Autodesk Fusion 360 part; units mm, degrees
(part 2 of 6)
  spline S13 degree 5 poles (-24.4636, 3.0462) (-24.4632, 3.0438) (-24.4623, 3.0389) (-24.4609, 3.0317) (-24.4591, 3.022) (-24.4568, 3.0099) (-24.4544, 2.9979) (-24.4519, 2.9859) (-24.4494, 2.9739) (-24.4468, 2.962) (-24.4442, 2.9501) (-24.4415, 2.9383) (-24.4387, 2.9265) (-24.4359, 2.9147) (-24.4331, 2.903) (-24.4301, 2.8914) (-24.4271, 2.8797) (-24.4241, 2.8681) (-24.421, 2.8566) (-24.4178, 2.8451) (-24.4146, 2.8336) (-24.4113, 2.8222) (-24.4079, 2.8108) (-24.4045, 2.7995) (-24.4011, 2.7882) (-24.3975, 2.777) (-24.3939, 2.7658) (-24.3903, 2.7547) (-24.3866, 2.7436) (-24.3828, 2.7325) (-24.379, 2.7215) (-24.3751, 2.7106) (-24.3711, 2.6997) (-24.3671, 2.6888) (-24.363, 2.678) (-24.3588, 2.6673) (-24.3546, 2.6566) (-24.3504, 2.646) (-24.346, 2.6354) (-24.3416, 2.6249) (-24.3372, 2.6144) (-24.3326, 2.604) (-24.328, 2.5936) (-24.3234, 2.5834) (-24.3186, 2.5731) (-24.3138, 2.5629) (-24.309, 2.5528) (-24.304, 2.5428) (-24.299, 2.5328) (-24.294, 2.5229) (-24.2888, 2.513) (-24.2836, 2.5032) (-24.2783, 2.4935) (-24.2729, 2.4839) (-24.2675, 2.4743) (-24.262, 2.4648) (-24.2564, 2.4554) (-24.2507, 2.446) (-24.245, 2.4368) (-24.2392, 2.4276) (-24.2333, 2.4185) (-24.2273, 2.4095) (-24.2211, 2.4006) (-24.2149, 2.3919) (-24.2085, 2.3832) (-24.2021, 2.3747) (-24.1956, 2.3662) (-24.1891, 2.3577) (-24.1825, 2.3494) (-24.1757, 2.3412) (-24.1687, 2.3333) (-24.1629, 2.3272) (-24.1583, 2.3228) (-24.1552, 2.32) (-24.1536, 2.3186) knots -1 -1 -1 -1 -1 -1 -0.98571429 -0.97142857 -0.95714286 -0.94285714 -0.92857143 -0.91428571 -0.9 -0.88571429 -0.87142857 -0.85714286 -0.84285714 -0.82857143 -0.81428571 -0.8 -0.78571429 -0.77142857 -0.75714286 -0.74285714 -0.72857143 -0.71428571 -0.7 -0.68571429 -0.67142857 -0.65714286 -0.64285714 -0.62857143 -0.61428571 -0.6 -0.58571429 -0.57142857 -0.55714286 -0.54285714 -0.52857143 -0.51428571 -0.5 -0.48571429 -0.47142857 -0.45714286 -0.44285714 -0.42857143 -0.41428571 -0.4 -0.38571429 -0.37142857 -0.35714286 -0.34285714 -0.32857143 -0.31428571 -0.3 -0.28571429 -0.27142857 -0.25714286 -0.24285714 -0.22857143 -0.21428571 -0.2 -0.18571429 -0.17142857 -0.15714286 -0.14285714 -0.12857143 -0.11428571 -0.1 -0.08571429 -0.07142857 -0.05714286 -0.04285714 -0.02857143 -0.01428571 0 0 0 0 0 0
  line L13 (-24.1536, 2.3186) -> (-24.0344, 2.2145)
  arc A27 (-24.0078, 1.9414) -> (-24.0344, 2.2145) centre (-24.166, 2.0639) ccw
  arc A28 (-24.0078, 1.9414) -> (-24.1214, 1.7852) centre (-21.5, 0) ccw
  arc A29 (-24.3893, 1.726) -> (-24.1214, 1.7852) centre (-24.2867, 1.8977) ccw
  line L14 (-24.3893, 1.726) -> (-24.5251, 1.8072)
  spline S14 degree 5 poles (-24.5251, 1.8072) (-24.527, 1.8083) (-24.5306, 1.8104) (-24.5362, 1.8134) (-24.5438, 1.8171) (-24.5535, 1.8213) (-24.5633, 1.8252) (-24.5733, 1.8289) (-24.5833, 1.8325) (-24.5934, 1.8361) (-24.6036, 1.8395) (-24.6137, 1.8429) (-24.624, 1.8461) (-24.6343, 1.8492) (-24.6447, 1.8522) (-24.6552, 1.855) (-24.6658, 1.8577) (-24.6764, 1.8602) (-24.687, 1.8627) (-24.6977, 1.8651) (-24.7084, 1.8674) (-24.7192, 1.8697) (-24.73, 1.8718) (-24.7409, 1.8738) (-24.7518, 1.8758) (-24.7628, 1.8776) (-24.7738, 1.8794) (-24.7848, 1.881) (-24.7959, 1.8826) (-24.807, 1.8841) (-24.8182, 1.8855) (-24.8294, 1.8869) (-24.8406, 1.8881) (-24.8519, 1.8893) (-24.8632, 1.8904) (-24.8745, 1.8914) (-24.8859, 1.8923) (-24.8973, 1.8932) (-24.9087, 1.894) (-24.9202, 1.8947) (-24.9317, 1.8953) (-24.9432, 1.8959) (-24.9548, 1.8963) (-24.9664, 1.8967) (-24.978, 1.8971) (-24.9896, 1.8973) (-25.0013, 1.8975) (-25.013, 1.8976) (-25.0247, 1.8976) (-25.0365, 1.8976) (-25.0482, 1.8975) (-25.06, 1.8973) (-25.0719, 1.897) (-25.0837, 1.8967) (-25.0956, 1.8963) (-25.1075, 1.8958) (-25.1194, 1.8953) (-25.1313, 1.8947) (-25.1433, 1.894) (-25.1553, 1.8932) (-25.1673, 1.8924) (-25.1793, 1.8915) (-25.1914, 1.8906) (-25.2035, 1.8895) (-25.2156, 1.8884) (-25.2277, 1.8873) (-25.2398, 1.8861) (-25.2519, 1.8848) (-25.2641, 1.8834) (-25.2763, 1.8819) (-25.2885, 1.8804) (-25.2983, 1.8792) (-25.3056, 1.8782) (-25.3105, 1.8776) (-25.3129, 1.8772) knots 0 0 0 0 0 0 0.01428571 0.02857143 0.04285714 0.05714286 0.07142857 0.08571429 0.1 0.11428571 0.12857143 0.14285714 0.15714286 0.17142857 0.18571429 0.2 0.21428571 0.22857143 0.24285714 0.25714286 0.27142857 0.28571429 0.3 0.31428571 0.32857143 0.34285714 0.35714286 0.37142857 0.38571429 0.4 0.41428571 0.42857143 0.44285714 0.45714286 0.47142857 0.48571429 0.5 0.51428571 0.52857143 0.54285714 0.55714286 0.57142857 0.58571429 0.6 0.61428571 0.62857143 0.64285714 0.65714286 0.67142857 0.68571429 0.7 0.71428571 0.72857143 0.74285714 0.75714286 0.77142857 0.78571429 0.8 0.81428571 0.82857143 0.84285714 0.85714286 0.87142857 0.88571429 0.9 0.91428571 0.92857143 0.94285714 0.95714286 0.97142857 0.98571429 1 1 1 1 1 1
  arc A30 (-25.3129, 1.8772) -> (-25.4464, 1.5775) centre (-21.5, 0) ccw
  spline S15 degree 5 poles (-25.4464, 1.5775) (-25.445, 1.5754) (-25.4422, 1.5713) (-25.438, 1.5652) (-25.4324, 1.5571) (-25.4254, 1.5471) (-25.4183, 1.537) (-25.4112, 1.5271) (-25.404, 1.5172) (-25.3968, 1.5074) (-25.3896, 1.4976) (-25.3823, 1.4879) (-25.375, 1.4782) (-25.3676, 1.4686) (-25.3603, 1.4591) (-25.3528, 1.4496) (-25.3454, 1.4402) (-25.3379, 1.4308) (-25.3303, 1.4216) (-25.3228, 1.4123) (-25.3151, 1.4032) (-25.3075, 1.3941) (-25.2998, 1.3851) (-25.2921, 1.3761) (-25.2843, 1.3672) (-25.2765, 1.3584) (-25.2687, 1.3496) (-25.2608, 1.3409) (-25.2529, 1.3323) (-25.245, 1.3237) (-25.237, 1.3153) (-25.229, 1.3068) (-25.2209, 1.2985) (-25.2129, 1.2902) (-25.2047, 1.282) (-25.1966, 1.2739) (-25.1884, 1.2659) (-25.1802, 1.2579) (-25.1719, 1.25) (-25.1636, 1.2422) (-25.1553, 1.2344) (-25.1469, 1.2267) (-25.1385, 1.2192) (-25.13, 1.2116) (-25.1215, 1.2042) (-25.113, 1.1969) (-25.1045, 1.1896) (-25.0959, 1.1824) (-25.0872, 1.1753) (-25.0786, 1.1683) (-25.0699, 1.1614) (-25.0611, 1.1546) (-25.0523, 1.1479) (-25.0435, 1.1413) (-25.0346, 1.1348) (-25.0257, 1.1283) (-25.0168, 1.122) (-25.0078, 1.1157) (-24.9988, 1.1096) (-24.9898, 1.1036) (-24.9807, 1.0976) (-24.9715, 1.0919) (-24.9623, 1.0863) (-24.953, 1.0808) (-24.9437, 1.0755) (-24.9344, 1.0703) (-24.925, 1.0652) (-24.9156, 1.0601) (-24.9062, 1.0552) (-24.8967, 1.0505) (-24.887, 1.0461) (-24.8792, 1.0429) (-24.8733, 1.0408) (-24.8693, 1.0395) (-24.8672, 1.0389) knots -1 -1 -1 -1 -1 -1 -0.98571429 -0.97142857 -0.95714286 -0.94285714 -0.92857143 -0.91428571 -0.9 -0.88571429 -0.87142857 -0.85714286 -0.84285714 -0.82857143 -0.81428571 -0.8 -0.78571429 -0.77142857 -0.75714286 -0.74285714 -0.72857143 -0.71428571 -0.7 -0.68571429 -0.67142857 -0.65714286 -0.64285714 -0.62857143 -0.61428571 -0.6 -0.58571429 -0.57142857 -0.55714286 -0.54285714 -0.52857143 -0.51428571 -0.5 -0.48571429 -0.47142857 -0.45714286 -0.44285714 -0.42857143 -0.41428571 -0.4 -0.38571429 -0.37142857 -0.35714286 -0.34285714 -0.32857143 -0.31428571 -0.3 -0.28571429 -0.27142857 -0.25714286 -0.24285714 -0.22857143 -0.21428571 -0.2 -0.18571429 -0.17142857 -0.15714286 -0.14285714 -0.12857143 -0.11428571 -0.1 -0.08571429 -0.07142857 -0.05714286 -0.04285714 -0.02857143 -0.01428571 0 0 0 0 0 0
  line L15 (-24.8672, 1.0389) -> (-24.716, 0.9922)
  arc A31 (-24.5807, 0.7536) -> (-24.716, 0.9922) centre (-24.7749, 0.8011) ccw
  arc A32 (-24.5807, 0.7536) -> (-24.6208, 0.5646) centre (-21.5, 0) ccw
  arc A33 (-24.8415, 0.4016) -> (-24.6208, 0.5646) centre (-24.8176, 0.6002) ccw
  line L16 (-24.8415, 0.4016) -> (-24.9987, 0.4205)
  spline S16 degree 5 poles (-24.9987, 0.4205) (-25.0008, 0.4208) (-25.005, 0.4212) (-25.0113, 0.4217) (-25.0197, 0.422) (-25.0303, 0.4219) (-25.0409, 0.4214) (-25.0515, 0.4208) (-25.0621, 0.42) (-25.0728, 0.4191) (-25.0834, 0.4181) (-25.0941, 0.4171) (-25.1048, 0.4159) (-25.1155, 0.4145) (-25.1262, 0.413) (-25.1369, 0.4113) (-25.1476, 0.4094) (-25.1584, 0.4075) (-25.1691, 0.4054) (-25.1799, 0.4033) (-25.1906, 0.401) (-25.2013, 0.3987) (-25.2121, 0.3962) (-25.2229, 0.3936) (-25.2336, 0.391) (-25.2444, 0.3882) (-25.2552, 0.3853) (-25.2659, 0.3824) (-25.2767, 0.3793) (-25.2875, 0.3761) (-25.2982, 0.3729) (-25.309, 0.3696) (-25.3198, 0.3661) (-25.3305, 0.3626) (-25.3413, 0.359) (-25.3521, 0.3554) (-25.3629, 0.3516) (-25.3736, 0.3477) (-25.3844, 0.3438) (-25.3951, 0.3398) (-25.4059, 0.3357) (-25.4167, 0.3315) (-25.4274, 0.3272) (-25.4381, 0.3229) (-25.4489, 0.3184) (-25.4596, 0.3139) (-25.4704, 0.3093) (-25.4811, 0.3047) (-25.4918, 0.2999) (-25.5025, 0.2951) (-25.5132, 0.2902) (-25.5239, 0.2853) (-25.5346, 0.2802) (-25.5453, 0.2751) (-25.556, 0.2699) (-25.5667, 0.2646) (-25.5774, 0.2593) (-25.588, 0.2539) (-25.5987, 0.2484) (-25.6093, 0.2428) (-25.62, 0.2372) (-25.6306, 0.2315) (-25.6412, 0.2257) (-25.6518, 0.2199) (-25.6624, 0.2139) (-25.673, 0.2079) (-25.6836, 0.2019) (-25.6942, 0.1958) (-25.7047, 0.1896) (-25.7153, 0.1833) (-25.7258, 0.177) (-25.7342, 0.1718) (-25.7405, 0.168) (-25.7447, 0.1654) (-25.7468, 0.1641) knots 0 0 0 0 0 0 0.01428571 0.02857143 0.04285714 0.05714286 0.07142857 0.08571429 0.1 0.11428571 0.12857143 0.14285714 0.15714286 0.17142857 0.18571429 0.2 0.21428571 0.22857143 0.24285714 0.25714286 0.27142857 0.28571429 0.3 0.31428571 0.32857143 0.34285714 0.35714286 0.37142857 0.38571429 0.4 0.41428571 0.42857143 0.44285714 0.45714286 0.47142857 0.48571429 0.5 0.51428571 0.52857143 0.54285714 0.55714286 0.57142857 0.58571429 0.6 0.61428571 0.62857143 0.64285714 0.65714286 0.67142857 0.68571429 0.7 0.71428571 0.72857143 0.74285714 0.75714286 0.77142857 0.78571429 0.8 0.81428571 0.82857143 0.84285714 0.85714286 0.87142857 0.88571429 0.9 0.91428571 0.92857143 0.94285714 0.95714286 0.97142857 0.98571429 1 1 1 1 1 1
  arc A34 (-25.7468, 0.1641) -> (-25.7468, -0.1641) centre (-21.5, 0) ccw
  spline S17 degree 5 poles (-25.7468, -0.1641) (-25.7447, -0.1654) (-25.7405, -0.168) (-25.7342, -0.1718) (-25.7258, -0.177) (-25.7153, -0.1833) (-25.7047, -0.1896) (-25.6942, -0.1958) (-25.6836, -0.2019) (-25.673, -0.2079) (-25.6624, -0.2139) (-25.6518, -0.2199) (-25.6412, -0.2257) (-25.6306, -0.2315) (-25.62, -0.2372) (-25.6093, -0.2428) (-25.5987, -0.2484) (-25.588, -0.2539) (-25.5774, -0.2593) (-25.5667, -0.2646) (-25.556, -0.2699) (-25.5453, -0.2751) (-25.5346, -0.2802) (-25.5239, -0.2853) (-25.5132, -0.2902) (-25.5025, -0.2951) (-25.4918, -0.2999) (-25.4811, -0.3047) (-25.4704, -0.3093) (-25.4596, -0.3139) (-25.4489, -0.3184) (-25.4381, -0.3229) (-25.4274, -0.3272) (-25.4167, -0.3315) (-25.4059, -0.3357) (-25.3951, -0.3398) (-25.3844, -0.3438) (-25.3736, -0.3477) (-25.3629, -0.3516) (-25.3521, -0.3554) (-25.3413, -0.359) (-25.3305, -0.3626) (-25.3198, -0.3661) (-25.309, -0.3696) (-25.2982, -0.3729) (-25.2875, -0.3761) (-25.2767, -0.3793) (-25.2659, -0.3824) (-25.2552, -0.3853) (-25.2444, -0.3882) (-25.2336, -0.391) (-25.2229, -0.3936) (-25.2121, -0.3962) (-25.2013, -0.3987) (-25.1906, -0.401) (-25.1799, -0.4033) (-25.1691, -0.4054) (-25.1584, -0.4075) (-25.1476, -0.4094) (-25.1369, -0.4113) (-25.1262, -0.413) (-25.1155, -0.4145) (-25.1048, -0.4159) (-25.0941, -0.4171) (-25.0834, -0.4181) (-25.0728, -0.4191) (-25.0621, -0.42) (-25.0515, -0.4208) (-25.0409, -0.4214) (-25.0303, -0.4219) (-25.0197, -0.422) (-25.0113, -0.4217) (-25.005, -0.4212) (-25.0008, -0.4208) (-24.9987, -0.4205) knots -1 -1 -1 -1 -1 -1 -0.98571429 -0.97142857 -0.95714286 -0.94285714 -0.92857143 -0.91428571 -0.9 -0.88571429 -0.87142857 -0.85714286 -0.84285714 -0.82857143 -0.81428571 -0.8 -0.78571429 -0.77142857 -0.75714286 -0.74285714 -0.72857143 -0.71428571 -0.7 -0.68571429 -0.67142857 -0.65714286 -0.64285714 -0.62857143 -0.61428571 -0.6 -0.58571429 -0.57142857 -0.55714286 -0.54285714 -0.52857143 -0.51428571 -0.5 -0.48571429 -0.47142857 -0.45714286 -0.44285714 -0.42857143 -0.41428571 -0.4 -0.38571429 -0.37142857 -0.35714286 -0.34285714 -0.32857143 -0.31428571 -0.3 -0.28571429 -0.27142857 -0.25714286 -0.24285714 -0.22857143 -0.21428571 -0.2 -0.18571429 -0.17142857 -0.15714286 -0.14285714 -0.12857143 -0.11428571 -0.1 -0.08571429 -0.07142857 -0.05714286 -0.04285714 -0.02857143 -0.01428571 0 0 0 0 0 0
  line L17 (-24.9987, -0.4205) -> (-24.8415, -0.4016)
  arc A35 (-24.6208, -0.5646) -> (-24.8415, -0.4016) centre (-24.8176, -0.6002) ccw
  arc A36 (-24.6208, -0.5646) -> (-24.5807, -0.7536) centre (-21.5, 0) ccw
  arc A37 (-24.716, -0.9922) -> (-24.5807, -0.7536) centre (-24.7749, -0.8011) ccw
  line L18 (-24.716, -0.9922) -> (-24.8672, -1.0389)
  spline S18 degree 5 poles (-24.8672, -1.0389) (-24.8693, -1.0395) (-24.8733, -1.0408) (-24.8792, -1.0429) (-24.887, -1.0461) (-24.8967, -1.0505) (-24.9062, -1.0552) (-24.9156, -1.0601) (-24.925, -1.0652) (-24.9344, -1.0703) (-24.9437, -1.0755) (-24.953, -1.0808) (-24.9623, -1.0863) (-24.9715, -1.0919) (-24.9807, -1.0976) (-24.9898, -1.1036) (-24.9988, -1.1096) (-25.0078, -1.1157) (-25.0168, -1.122) (-25.0257, -1.1283) (-25.0346, -1.1348) (-25.0435, -1.1413) (-25.0523, -1.1479) (-25.0611, -1.1546) (-25.0699, -1.1614) (-25.0786, -1.1683) (-25.0872, -1.1753) (-25.0959, -1.1824) (-25.1045, -1.1896) (-25.113, -1.1969) (-25.1215, -1.2042) (-25.13, -1.2116) (-25.1385, -1.2192) (-25.1469, -1.2267) (-25.1553, -1.2344) (-25.1636, -1.2422) (-25.1719, -1.25) (-25.1802, -1.2579) (-25.1884, -1.2659) (-25.1966, -1.2739) (-25.2047, -1.282) (-25.2129, -1.2902) (-25.2209, -1.2985) (-25.229, -1.3068) (-25.237, -1.3153) (-25.245, -1.3237) (-25.2529, -1.3323) (-25.2608, -1.3409) (-25.2687, -1.3496) (-25.2765, -1.3584) (-25.2843, -1.3672) (-25.2921, -1.3761) (-25.2998, -1.3851) (-25.3075, -1.3941) (-25.3151, -1.4032) (-25.3228, -1.4123) (-25.3303, -1.4216) (-25.3379, -1.4308) (-25.3454, -1.4402) (-25.3528, -1.4496) (-25.3603, -1.4591) (-25.3676, -1.4686) (-25.375, -1.4782) (-25.3823, -1.4879) (-25.3896, -1.4976) (-25.3968, -1.5074) (-25.404, -1.5172) (-25.4112, -1.5271) (-25.4183, -1.537) (-25.4254, -1.5471) (-25.4324, -1.5571) (-25.438, -1.5652) (-25.4422, -1.5713) (-25.445, -1.5754) (-25.4464, -1.5775) knots 0 0 0 0 0 0 0.01428571 0.02857143 0.04285714 0.05714286 0.07142857 0.08571429 0.1 0.11428571 0.12857143 0.14285714 0.15714286 0.17142857 0.18571429 0.2 0.21428571 0.22857143 0.24285714 0.25714286 0.27142857 0.28571429 0.3 0.31428571 0.32857143 0.34285714 0.35714286 0.37142857 0.38571429 0.4 0.41428571 0.42857143 0.44285714 0.45714286 0.47142857 0.48571429 0.5 0.51428571 0.52857143 0.54285714 0.55714286 0.57142857 0.58571429 0.6 0.61428571 0.62857143 0.64285714 0.65714286 0.67142857 0.68571429 0.7 0.71428571 0.72857143 0.74285714 0.75714286 0.77142857 0.78571429 0.8 0.81428571 0.82857143 0.84285714 0.85714286 0.87142857 0.88571429 0.9 0.91428571 0.92857143 0.94285714 0.95714286 0.97142857 0.98571429 1 1 1 1 1 1
  arc A38 (-25.4464, -1.5775) -> (-25.3129, -1.8772) centre (-21.5, 0) ccw
  spline S19 degree 5 poles (-25.3129, -1.8772) (-25.3105, -1.8776) (-25.3056, -1.8782) (-25.2983, -1.8792) (-25.2885, -1.8804) (-25.2763, -1.8819) (-25.2641, -1.8834) (-25.2519, -1.8848) (-25.2398, -1.8861) (-25.2277, -1.8873) (-25.2156, -1.8884) (-25.2035, -1.8895) (-25.1914, -1.8906) (-25.1793, -1.8915) (-25.1673, -1.8924) (-25.1553, -1.8932) (-25.1433, -1.894) (-25.1313, -1.8947) (-25.1194, -1.8953) (-25.1075, -1.8958) (-25.0956, -1.8963) (-25.0837, -1.8967) (-25.0719, -1.897) (-25.06, -1.8973) (-25.0482, -1.8975) (-25.0365, -1.8976) (-25.0247, -1.8976) (-25.013, -1.8976) (-25.0013, -1.8975) (-24.9896, -1.8973) (-24.978, -1.8971) (-24.9664, -1.8967) (-24.9548, -1.8963) (-24.9432, -1.8959) (-24.9317, -1.8953) (-24.9202, -1.8947) (-24.9087, -1.894) (-24.8973, -1.8932) (-24.8859, -1.8923) (-24.8745, -1.8914) (-24.8632, -1.8904) (-24.8519, -1.8893) (-24.8406, -1.8881) (-24.8294, -1.8869) (-24.8182, -1.8855) (-24.807, -1.8841) (-24.7959, -1.8826) (-24.7848, -1.881) (-24.7738, -1.8794) (-24.7628, -1.8776) (-24.7518, -1.8758) (-24.7409, -1.8738) (-24.73, -1.8718) (-24.7192, -1.8697) (-24.7084, -1.8674) (-24.6977, -1.8651) (-24.687, -1.8627) (-24.6764, -1.8602) (-24.6658, -1.8577) (-24.6552, -1.855) (-24.6447, -1.8522) (-24.6343, -1.8492) (-24.624, -1.8461) (-24.6137, -1.8429) (-24.6036, -1.8395) (-24.5934, -1.8361) (-24.5833, -1.8325) (-24.5733, -1.8289) (-24.5633, -1.8252) (-24.5535, -1.8213) (-24.5438, -1.8171) (-24.5362, -1.8134) (-24.5306, -1.8104) (-24.527, -1.8083) (-24.5251, -1.8072) knots -1 -1 -1 -1 -1 -1 -0.98571429 -0.97142857 -0.95714286 -0.94285714 -0.92857143 -0.91428571 -0.9 -0.88571429 -0.87142857 -0.85714286 -0.84285714 -0.82857143 -0.81428571 -0.8 -0.78571429 -0.77142857 -0.75714286 -0.74285714 -0.72857143 -0.71428571 -0.7 -0.68571429 -0.67142857 -0.65714286 -0.64285714 -0.62857143 -0.61428571 -0.6 -0.58571429 -0.57142857 -0.55714286 -0.54285714 -0.52857143 -0.51428571 -0.5 -0.48571429 -0.47142857 -0.45714286 -0.44285714 -0.42857143 -0.41428571 -0.4 -0.38571429 -0.37142857 -0.35714286 -0.34285714 -0.32857143 -0.31428571 -0.3 -0.28571429 -0.27142857 -0.25714286 -0.24285714 -0.22857143 -0.21428571 -0.2 -0.18571429 -0.17142857 -0.15714286 -0.14285714 -0.12857143 -0.11428571 -0.1 -0.08571429 -0.07142857 -0.05714286 -0.04285714 -0.02857143 -0.01428571 0 0 0 0 0 0
  line L19 (-24.5251, -1.8072) -> (-24.3893, -1.726)
  arc A39 (-24.1214, -1.7852) -> (-24.3893, -1.726) centre (-24.2867, -1.8977) ccw
  arc A40 (-24.1214, -1.7852) -> (-24.0078, -1.9414) centre (-21.5, 0) ccw
  arc A41 (-24.0344, -2.2145) -> (-24.0078, -1.9414) centre (-24.166, -2.0639) ccw
  line L20 (-24.0344, -2.2145) -> (-24.1536, -2.3186)
  spline S20 degree 5 poles (-24.1536, -2.3186) (-24.1552, -2.32) (-24.1583, -2.3228) (-24.1629, -2.3272) (-24.1687, -2.3333) (-24.1757, -2.3412) (-24.1825, -2.3494) (-24.1891, -2.3577) (-24.1956, -2.3662) (-24.2021, -2.3747) (-24.2085, -2.3832) (-24.2149, -2.3919) (-24.2211, -2.4006) (-24.2273, -2.4095) (-24.2333, -2.4185) (-24.2392, -2.4276) (-24.245, -2.4368) (-24.2507, -2.446) (-24.2564, -2.4554) (-24.262, -2.4648) (-24.2675, -2.4743) (-24.2729, -2.4839) (-24.2783, -2.4935) (-24.2836, -2.5032) (-24.2888, -2.513) (-24.294, -2.5229) (-24.299, -2.5328) (-24.304, -2.5428) (-24.309, -2.5528) (-24.3138, -2.5629) (-24.3186, -2.5731) (-24.3234, -2.5834) (-24.328, -2.5936) (-24.3326, -2.604) (-24.3372, -2.6144) (-24.3416, -2.6249) (-24.346, -2.6354) (-24.3504, -2.646) (-24.3546, -2.6566) (-24.3588, -2.6673) (-24.363, -2.678) (-24.3671, -2.6888) (-24.3711, -2.6997) (-24.3751, -2.7106) (-24.379, -2.7215) (-24.3828, -2.7325) (-24.3866, -2.7436) (-24.3903, -2.7547) (-24.3939, -2.7658) (-24.3975, -2.777) (-24.4011, -2.7882) (-24.4045, -2.7995) (-24.4079, -2.8108) (-24.4113, -2.8222) (-24.4146, -2.8336) (-24.4178, -2.8451) (-24.421, -2.8566) (-24.4241, -2.8681) (-24.4271, -2.8797) (-24.4301, -2.8914) (-24.4331, -2.903) (-24.4359, -2.9147) (-24.4387, -2.9265) (-24.4415, -2.9383) (-24.4442, -2.9501) (-24.4468, -2.962) (-24.4494, -2.9739) (-24.4519, -2.9859) (-24.4544, -2.9979) (-24.4568, -3.0099) (-24.4591, -3.022) (-24.4609, -3.0317) (-24.4623, -3.0389) (-24.4632, -3.0438) (-24.4636, -3.0462) knots 0 0 0 0 0 0 0.01428571 0.02857143 0.04285714 0.05714286 0.07142857 0.08571429 0.1 0.11428571 0.12857143 0.14285714 0.15714286 0.17142857 0.18571429 0.2 0.21428571 0.22857143 0.24285714 0.25714286 0.27142857 0.28571429 0.3 0.31428571 0.32857143 0.34285714 0.35714286 0.37142857 0.38571429 0.4 0.41428571 0.42857143 0.44285714 0.45714286 0.47142857 0.48571429 0.5 0.51428571 0.52857143 0.54285714 0.55714286 0.57142857 0.58571429 0.6 0.61428571 0.62857143 0.64285714 0.65714286 0.67142857 0.68571429 0.7 0.71428571 0.72857143 0.74285714 0.75714286 0.77142857 0.78571429 0.8 0.81428571 0.82857143 0.84285714 0.85714286 0.87142857 0.88571429 0.9 0.91428571 0.92857143 0.94285714 0.95714286 0.97142857 0.98571429 1 1 1 1 1 1
  arc A42 (-24.4636, -3.0462) -> (-24.2198, -3.2658) centre (-21.5, 0) ccw
  spline S21 degree 5 poles (-24.2198, -3.2658) (-24.2174, -3.2651) (-24.2127, -3.2637) (-24.2056, -3.2616) (-24.1961, -3.2588) (-24.1844, -3.2552) (-24.1726, -3.2516) (-24.161, -3.2479) (-24.1493, -3.2441) (-24.1378, -3.2403) (-24.1262, -3.2364) (-24.1147, -3.2325) (-24.1033, -3.2285) (-24.0919, -3.2245) (-24.0805, -3.2204) (-24.0692, -3.2163) (-24.058, -3.2121) (-24.0468, -3.2079) (-24.0356, -3.2036) (-24.0245, -3.1992) (-24.0134, -3.1948) (-24.0024, -3.1903) (-23.9915, -3.1858) (-23.9806, -3.1812) (-23.9697, -3.1766) (-23.9589, -3.1719) (-23.9482, -3.1672) (-23.9375, -3.1624) (-23.9268, -3.1575) (-23.9162, -3.1526) (-23.9057, -3.1477) (-23.8952, -3.1426) (-23.8848, -3.1376) (-23.8744, -3.1324) (-23.8641, -3.1272) (-23.8539, -3.122) (-23.8437, -3.1167) (-23.8335, -3.1113) (-23.8235, -3.1059) (-23.8135, -3.1004) (-23.8035, -3.0949) (-23.7936, -3.0893) (-23.7838, -3.0836) (-23.7741, -3.0779) (-23.7644, -3.0722) (-23.7548, -3.0663) (-23.7452, -3.0604) (-23.7357, -3.0545) (-23.7263, -3.0485) (-23.717, -3.0424) (-23.7077, -3.0362) (-23.6985, -3.03) (-23.6894, -3.0237) (-23.6804, -3.0174) (-23.6715, -3.011) (-23.6626, -3.0045) (-23.6538, -2.998) (-23.6451, -2.9914) (-23.6365, -2.9847) (-23.6279, -2.978) (-23.6195, -2.9711) (-23.6112, -2.9642) (-23.603, -2.9572) (-23.595, -2.95) (-23.587, -2.9428) (-23.5792, -2.9355) (-23.5714, -2.9282) (-23.5637, -2.9208) (-23.5561, -2.9134) (-23.5487, -2.9058) (-23.5415, -2.898) (-23.5361, -2.8916) (-23.5322, -2.8865) (-23.5298, -2.8831) (-23.5285, -2.8814) knots -1 -1 -1 -1 -1 -1 -0.98571429 -0.97142857 -0.95714286 -0.94285714 -0.92857143 -0.91428571 -0.9 -0.88571429 -0.87142857 -0.85714286 -0.84285714 -0.82857143 -0.81428571 -0.8 -0.78571429 -0.77142857 -0.75714286 -0.74285714 -0.72857143 -0.71428571 -0.7 -0.68571429 -0.67142857 -0.65714286 -0.64285714 -0.62857143 -0.61428571 -0.6 -0.58571429 -0.57142857 -0.55714286 -0.54285714 -0.52857143 -0.51428571 -0.5 -0.48571429 -0.47142857 -0.45714286 -0.44285714 -0.42857143 -0.41428571 -0.4 -0.38571429 -0.37142857 -0.35714286 -0.34285714 -0.32857143 -0.31428571 -0.3 -0.28571429 -0.27142857 -0.25714286 -0.24285714 -0.22857143 -0.21428571 -0.2 -0.18571429 -0.17142857 -0.15714286 -0.14285714 -0.12857143 -0.11428571 -0.1 -0.08571429 -0.07142857 -0.05714286 -0.04285714 -0.02857143 -0.01428571 0 0 0 0 0 0
  line L21 (-23.5285, -2.8814) -> (-23.4374, -2.752)
  arc A43 (-23.1687, -2.697) -> (-23.4374, -2.752) centre (-23.2739, -2.8671) ccw
  arc A44 (-23.1687, -2.697) -> (-23.0014, -2.7936) centre (-21.5, 0) ccw
  arc A45 (-22.9146, -3.0539) -> (-23.0014, -2.7936) centre (-23.096, -2.9698) ccw
  line L22 (-22.9146, -3.0539) -> (-22.9811, -3.1975)
  spline S22 degree 5 poles (-22.9811, -3.1975) (-22.982, -3.1994) (-22.9837, -3.2032) (-22.9861, -3.2091) (-22.989, -3.217) (-22.9922, -3.2271) (-22.995, -3.2373) (-22.9976, -3.2476) (-23.0002, -3.258) (-23.0026, -3.2684) (-23.005, -3.2788) (-23.0073, -3.2893) (-23.0095, -3.2999) (-23.0115, -3.3105) (-23.0133, -3.3211) (-23.015, -3.3318) (-23.0166, -3.3426) (-23.018, -3.3534) (-23.0194, -3.3643) (-23.0207, -3.3751) (-23.0218, -3.386) (-23.0229, -3.397) (-23.0239, -3.408) (-23.0248, -3.419) (-23.0256, -3.4301) (-23.0263, -3.4412) (-23.0269, -3.4523) (-23.0274, -3.4635) (-23.0278, -3.4746) (-23.0281, -3.4859) (-23.0284, -3.4971) (-23.0285, -3.5084) (-23.0286, -3.5197) (-23.0286, -3.531) (-23.0285, -3.5424) (-23.0283, -3.5537) (-23.0281, -3.5651) (-23.0277, -3.5766) (-23.0273, -3.588) (-23.0268, -3.5995) (-23.0262, -3.611) (-23.0256, -3.6225) (-23.0248, -3.6341) (-23.024, -3.6456) (-23.0231, -3.6572) (-23.0222, -3.6688) (-23.0211, -3.6804) (-23.02, -3.6921) (-23.0188, -3.7038) (-23.0175, -3.7154) (-23.0162, -3.7271) (-23.0148, -3.7389) (-23.0133, -3.7506) (-23.0117, -3.7623) (-23.0101, -3.7741) (-23.0084, -3.7859) (-23.0066, -3.7977) (-23.0047, -3.8095) (-23.0028, -3.8213) (-23.0008, -3.8332) (-22.9987, -3.845) (-22.9966, -3.8569) (-22.9944, -3.8688) (-22.9921, -3.8807) (-22.9897, -3.8926) (-22.9873, -3.9045) (-22.9848, -3.9164) (-22.9822, -3.9284) (-22.9796, -3.9403) (-22.9769, -3.9523) (-22.9741, -3.9643) (-22.9719, -3.9739) (-22.9701, -3.9811) (-22.969, -3.9859) (-22.9684, -3.9883) knots 0 0 0 0 0 0 0.01428571 0.02857143 0.04285714 0.05714286 0.07142857 0.08571429 0.1 0.11428571 0.12857143 0.14285714 0.15714286 0.17142857 0.18571429 0.2 0.21428571 0.22857143 0.24285714 0.25714286 0.27142857 0.28571429 0.3 0.31428571 0.32857143 0.34285714 0.35714286 0.37142857 0.38571429 0.4 0.41428571 0.42857143 0.44285714 0.45714286 0.47142857 0.48571429 0.5 0.51428571 0.52857143 0.54285714 0.55714286 0.57142857 0.58571429 0.6 0.61428571 0.62857143 0.64285714 0.65714286 0.67142857 0.68571429 0.7 0.71428571 0.72857143 0.74285714 0.75714286 0.77142857 0.78571429 0.8 0.81428571 0.82857143 0.84285714 0.85714286 0.87142857 0.88571429 0.9 0.91428571 0.92857143 0.94285714 0.95714286 0.97142857 0.98571429 1 1 1 1 1 1
  arc A46 (-22.9684, -3.9883) -> (-22.6563, -4.0897) centre (-21.5, 0) ccw
  spline S23 degree 5 poles (-22.6563, -4.0897) (-22.6544, -4.0881) (-22.6507, -4.0849) (-22.645, -4.0801) (-22.6376, -4.0737) (-22.6283, -4.0656) (-22.619, -4.0575) (-22.6099, -4.0494) (-22.6008, -4.0412) (-22.5918, -4.033) (-22.5828, -4.0248) (-22.5739, -4.0166) (-22.5651, -4.0083) (-22.5563, -4) (-22.5476, -3.9916) (-22.5389, -3.9832) (-22.5303, -3.9748) (-22.5218, -3.9664) (-22.5134, -3.9579) (-22.505, -3.9494) (-22.4967, -3.9409) (-22.4885, -3.9324) (-22.4803, -3.9238) (-22.4722, -3.9152) (-22.4641, -3.9065) (-22.4562, -3.8978) (-22.4483, -3.8891) (-22.4405, -3.8804) (-22.4327, -3.8716) (-22.425, -3.8628) (-22.4174, -3.854) (-22.4099, -3.8452) (-22.4024, -3.8363) (-22.3951, -3.8274) (-22.3878, -3.8185) (-22.3805, -3.8095) (-22.3734, -3.8005) (-22.3663, -3.7915) (-22.3593, -3.7824) (-22.3524, -3.7734) (-22.3456, -3.7643) (-22.3388, -3.7551) (-22.3321, -3.746) (-22.3256, -3.7368) (-22.3191, -3.7276) (-22.3127, -3.7183) (-22.3063, -3.7091) (-22.3001, -3.6998) (-22.2939, -3.6904) (-22.2879, -3.6811) (-22.2819, -3.6717) (-22.276, -3.6623) (-22.2703, -3.6529) (-22.2646, -3.6434) (-22.2591, -3.6339) (-22.2536, -3.6244) (-22.2482, -3.6148) (-22.243, -3.6052) (-22.2378, -3.5956) (-22.2327, -3.586) (-22.2278, -3.5763) (-22.223, -3.5666) (-22.2184, -3.5569) (-22.214, -3.5471) (-22.2097, -3.5373) (-22.2055, -3.5274) (-22.2013, -3.5176) (-22.1973, -3.5077) (-22.1934, -3.4978) (-22.1897, -3.4879) (-22.1863, -3.4778) (-22.184, -3.4697) (-22.1825, -3.4636) (-22.1816, -3.4595) (-22.1812, -3.4574) knots -1 -1 -1 -1 -1 -1 -0.98571429 -0.97142857 -0.95714286 -0.94285714 -0.92857143 -0.91428571 -0.9 -0.88571429 -0.87142857 -0.85714286 -0.84285714 -0.82857143 -0.81428571 -0.8 -0.78571429 -0.77142857 -0.75714286 -0.74285714 -0.72857143 -0.71428571 -0.7 -0.68571429 -0.67142857 -0.65714286 -0.64285714 -0.62857143 -0.61428571 -0.6 -0.58571429 -0.57142857 -0.55714286 -0.54285714 -0.52857143 -0.51428571 -0.5 -0.48571429 -0.47142857 -0.45714286 -0.44285714 -0.42857143 -0.41428571 -0.4 -0.38571429 -0.37142857 -0.35714286 -0.34285714 -0.32857143 -0.31428571 -0.3 -0.28571429 -0.27142857 -0.25714286 -0.24285714 -0.22857143 -0.21428571 -0.2 -0.18571429 -0.17142857 -0.15714286 -0.14285714 -0.12857143 -0.11428571 -0.1 -0.08571429 -0.07142857 -0.05714286 -0.04285714 -0.02857143 -0.01428571 0 0 0 0 0 0
  line L23 (-22.1812, -3.4574) -> (-22.1506, -3.3021)
  arc A47 (-21.9274, -3.1426) -> (-22.1506, -3.3021) centre (-21.9544, -3.3407) ccw
  arc A48 (-21.9274, -3.1426) -> (-21.7353, -3.1628) centre (-21.5, 0) ccw
  arc A49 (-21.5502, -3.3652) -> (-21.7353, -3.1628) centre (-21.7501, -3.3622) ccw
  line L24 (-21.5502, -3.3652) -> (-21.5525, -3.5235)
  spline S24 degree 5 poles (-21.5525, -3.5235) (-21.5526, -3.5256) (-21.5526, -3.5298) (-21.5524, -3.5361) (-21.5518, -3.5445) (-21.5506, -3.555) (-21.549, -3.5655) (-21.5472, -3.576) (-21.5453, -3.5865) (-21.5434, -3.597) (-21.5413, -3.6075) (-21.5391, -3.618) (-21.5368, -3.6285) (-21.5343, -3.639) (-21.5317, -3.6495) (-21.5289, -3.66) (-21.5259, -3.6705) (-21.5228, -3.6809) (-21.5197, -3.6914) (-21.5164, -3.7018) (-21.513, -3.7123) (-21.5096, -3.7227) (-21.506, -3.7332) (-21.5023, -3.7436) (-21.4986, -3.754) (-21.4947, -3.7645) (-21.4907, -3.7749) (-21.4866, -3.7853) (-21.4824, -3.7956) (-21.4782, -3.806) (-21.4738, -3.8164) (-21.4694, -3.8268) (-21.4649, -3.8371) (-21.4603, -3.8475) (-21.4555, -3.8578) (-21.4508, -3.8681) (-21.4459, -3.8784) (-21.4409, -3.8887) (-21.4359, -3.899) (-21.4307, -3.9093) (-21.4255, -3.9196) (-21.4203, -3.9298) (-21.4149, -3.9401) (-21.4094, -3.9503) (-21.4039, -3.9605) (-21.3983, -3.9708) (-21.3926, -3.9809) (-21.3869, -3.9911) (-21.381, -4.0013) (-21.3751, -4.0115) (-21.3691, -4.0216) (-21.3631, -4.0317) (-21.3569, -4.0418) (-21.3507, -4.0519) (-21.3444, -4.062) (-21.3381, -4.0721) (-21.3317, -4.0821) (-21.3252, -4.0922) (-21.3186, -4.1022) (-21.3119, -4.1122) (-21.3052, -4.1222) (-21.2984, -4.1322) (-21.2916, -4.1421) (-21.2847, -4.1521) (-21.2777, -4.162) (-21.2706, -4.1719) (-21.2635, -4.1818) (-21.2563, -4.1916) (-21.249, -4.2015) (-21.2417, -4.2113) (-21.2343, -4.2211) (-21.2283, -4.229) (-21.2238, -4.2349) (-21.2208, -4.2388) (-21.2192, -4.2407) knots 0 0 0 0 0 0 0.01428571 0.02857143 0.04285714 0.05714286 0.07142857 0.08571429 0.1 0.11428571 0.12857143 0.14285714 0.15714286 0.17142857 0.18571429 0.2 0.21428571 0.22857143 0.24285714 0.25714286 0.27142857 0.28571429 0.3 0.31428571 0.32857143 0.34285714 0.35714286 0.37142857 0.38571429 0.4 0.41428571 0.42857143 0.44285714 0.45714286 0.47142857 0.48571429 0.5 0.51428571 0.52857143 0.54285714 0.55714286 0.57142857 0.58571429 0.6 0.61428571 0.62857143 0.64285714 0.65714286 0.67142857 0.68571429 0.7 0.71428571 0.72857143 0.74285714 0.75714286 0.77142857 0.78571429 0.8 0.81428571 0.82857143 0.84285714 0.85714286 0.87142857 0.88571429 0.9 0.91428571 0.92857143 0.94285714 0.95714286 0.97142857 0.98571429 1 1 1 1 1 1
  arc A50 (-21.2192, -4.2407) -> (-20.8929, -4.2064) centre (-21.5, 0) ccw
  spline S25 degree 5 poles (-20.8929, -4.2064) (-20.8919, -4.2042) (-20.8897, -4.1997) (-20.8865, -4.1931) (-20.8823, -4.1842) (-20.8771, -4.173) (-20.872, -4.1619) (-20.8669, -4.1507) (-20.8619, -4.1396) (-20.857, -4.1284) (-20.8521, -4.1173) (-20.8474, -4.1061) (-20.8427, -4.0949) (-20.838, -4.0838) (-20.8335, -4.0726) (-20.829, -4.0614) (-20.8246, -4.0503) (-20.8202, -4.0391) (-20.8159, -4.0279) (-20.8117, -4.0168) (-20.8076, -4.0056) (-20.8036, -3.9944) (-20.7996, -3.9833) (-20.7957, -3.9721) (-20.7919, -3.9609) (-20.7881, -3.9498) (-20.7845, -3.9386) (-20.7809, -3.9274) (-20.7773, -3.9163) (-20.7739, -3.9051) (-20.7705, -3.894) (-20.7673, -3.8828) (-20.7641, -3.8717) (-20.7609, -3.8605) (-20.7579, -3.8494) (-20.7549, -3.8383) (-20.7521, -3.8272) (-20.7493, -3.816) (-20.7466, -3.8049) (-20.7439, -3.7938) (-20.7414, -3.7827) (-20.7389, -3.7717) (-20.7366, -3.7606) (-20.7343, -3.7495) (-20.7321, -3.7384) (-20.73, -3.7274) (-20.728, -3.7164) (-20.7261, -3.7053) (-20.7243, -3.6943) (-20.7225, -3.6833) (-20.7209, -3.6723) (-20.7194, -3.6613) (-20.7179, -3.6504) (-20.7166, -3.6394) (-20.7154, -3.6285) (-20.7143, -3.6175) (-20.7133, -3.6066) (-20.7124, -3.5957) (-20.7115, -3.5849) (-20.7108, -3.574) (-20.7102, -3.5632) (-20.7098, -3.5524) (-20.7096, -3.5416) (-20.7095, -3.5308) (-20.7096, -3.5201) (-20.7097, -3.5094) (-20.71, -3.4987) (-20.7103, -3.4881) (-20.7107, -3.4774) (-20.7114, -3.4668) (-20.7124, -3.4563) (-20.7136, -3.4479) (-20.7147, -3.4417) (-20.7156, -3.4376) (-20.7161, -3.4355) knots -1 -1 -1 -1 -1 -1 -0.98571429 -0.97142857 -0.95714286 -0.94285714 -0.92857143 -0.91428571 -0.9 -0.88571429 -0.87142857 -0.85714286 -0.84285714 -0.82857143 -0.81428571 -0.8 -0.78571429 -0.77142857 -0.75714286 -0.74285714 -0.72857143 -0.71428571 -0.7 -0.68571429 -0.67142857 -0.65714286 -0.64285714 -0.62857143 -0.61428571 -0.6 -0.58571429 -0.57142857 -0.55714286 -0.54285714 -0.52857143 -0.51428571 -0.5 -0.48571429 -0.47142857 -0.45714286 -0.44285714 -0.42857143 -0.41428571 -0.4 -0.38571429 -0.37142857 -0.35714286 -0.34285714 -0.32857143 -0.31428571 -0.3 -0.28571429 -0.27142857 -0.25714286 -0.24285714 -0.22857143 -0.21428571 -0.2 -0.18571429 -0.17142857 -0.15714286 -0.14285714 -0.12857143 -0.11428571 -0.1 -0.08571429 -0.07142857 -0.05714286 -0.04285714 -0.02857143 -0.01428571 0 0 0 0 0 0
  line L25 (-20.7161, -3.4355) -> (-20.7513, -3.2812)
  arc A51 (-20.6123, -3.0447) -> (-20.7513, -3.2812) centre (-20.5563, -3.2367) ccw
  arc A52 (-20.6123, -3.0447) -> (-20.4285, -2.985) centre (-21.5, 0) ccw
  arc A53 (-20.1771, -3.0947) -> (-20.4285, -2.985) centre (-20.361, -3.1733) ccw
  line L26 (-20.1771, -3.0947) -> (-20.1149, -3.2402)
  spline S26 degree 5 poles (-20.1149, -3.2402) (-20.114, -3.2421) (-20.1123, -3.246) (-20.1096, -3.2517) (-20.1056, -3.2591) (-20.1002, -3.2682) (-20.0945, -3.2772) (-20.0887, -3.2861) (-20.0826, -3.2949) (-20.0766, -3.3037) (-20.0704, -3.3124) (-20.0641, -3.3211) (-20.0578, -3.3298) (-20.0512, -3.3384) (-20.0445, -3.3469) (-20.0377, -3.3553) (-20.0308, -3.3637) (-20.0237, -3.372) (-20.0165, -3.3802) (-20.0093, -3.3885) (-20.002, -3.3967) (-19.9946, -3.4048) (-19.9871, -3.4129) (-19.9795, -3.4209) (-19.9718, -3.4289) (-19.964, -3.4368) (-19.9561, -3.4447) (-19.9482, -3.4526) (-19.9401, -3.4604) (-19.932, -3.4681) (-19.9238, -3.4758) (-19.9156, -3.4835) (-19.9072, -3.4911) (-19.8988, -3.4987) (-19.8903, -3.5062) (-19.8817, -3.5137) (-19.8731, -3.5211) (-19.8643, -3.5285) (-19.8555, -3.5359) (-19.8467, -3.5432) (-19.8377, -3.5504) (-19.8287, -3.5577) (-19.8197, -3.5648) (-19.8105, -3.572) (-19.8013, -3.5791) (-19.792, -3.5861) (-19.7827, -3.5931) (-19.7733, -3.6001) (-19.7638, -3.607) (-19.7543, -3.6139) (-19.7447, -3.6207) (-19.7351, -3.6275) (-19.7253, -3.6342) (-19.7156, -3.6409) (-19.7057, -3.6476) (-19.6958, -3.6542) (-19.6859, -3.6607) (-19.6758, -3.6673) (-19.6658, -3.6738) (-19.6556, -3.6802) (-19.6454, -3.6866) (-19.6352, -3.6929) (-19.6249, -3.6993) (-19.6145, -3.7055) (-19.6041, -3.7117) (-19.5936, -3.7179) (-19.583, -3.724) (-19.5724, -3.7301) (-19.5618, -3.7362) (-19.5511, -3.7422) (-19.5403, -3.7481) (-19.5317, -3.7529) (-19.5252, -3.7564) (-19.5208, -3.7587) (-19.5187, -3.7599) knots 0 0 0 0 0 0 0.01428571 0.02857143 0.04285714 0.05714286 0.07142857 0.08571429 0.1 0.11428571 0.12857143 0.14285714 0.15714286 0.17142857 0.18571429 0.2 0.21428571 0.22857143 0.24285714 0.25714286 0.27142857 0.28571429 0.3 0.31428571 0.32857143 0.34285714 0.35714286 0.37142857 0.38571429 0.4 0.41428571 0.42857143 0.44285714 0.45714286 0.47142857 0.48571429 0.5 0.51428571 0.52857143 0.54285714 0.55714286 0.57142857 0.58571429 0.6 0.61428571 0.62857143 0.64285714 0.65714286 0.67142857 0.68571429 0.7 0.71428571 0.72857143 0.74285714 0.75714286 0.77142857 0.78571429 0.8 0.81428571 0.82857143 0.84285714 0.85714286 0.87142857 0.88571429 0.9 0.91428571 0.92857143 0.94285714 0.95714286 0.97142857 0.98571429 1 1 1 1 1 1
  arc A54 (-19.5187, -3.7599) -> (-19.2345, -3.5958) centre (-21.5, 0) ccw
  spline S27 degree 5 poles (-19.2345, -3.5958) (-19.2344, -3.5934) (-19.2343, -3.5884) (-19.2341, -3.581) (-19.2339, -3.5712) (-19.2336, -3.5589) (-19.2335, -3.5466) (-19.2334, -3.5344) (-19.2334, -3.5222) (-19.2334, -3.51) (-19.2335, -3.4978) (-19.2337, -3.4857) (-19.2339, -3.4735) (-19.2342, -3.4615) (-19.2346, -3.4494) (-19.235, -3.4374) (-19.2356, -3.4254) (-19.2361, -3.4134) (-19.2368, -3.4015) (-19.2375, -3.3896) (-19.2383, -3.3777) (-19.2391, -3.3658) (-19.24, -3.354) (-19.241, -3.3422) (-19.242, -3.3305) (-19.2432, -3.3187) (-19.2443, -3.307) (-19.2456, -3.2954) (-19.2469, -3.2838) (-19.2483, -3.2722) (-19.2498, -3.2606) (-19.2513, -3.2491) (-19.2529, -3.2376) (-19.2546, -3.2262) (-19.2564, -3.2148) (-19.2582, -3.2034) (-19.2601, -3.1921) (-19.2621, -3.1808) (-19.2641, -3.1695) (-19.2662, -3.1583) (-19.2684, -3.1472) (-19.2707, -3.136) (-19.273, -3.1249) (-19.2754, -3.1139) (-19.2779, -3.1029) (-19.2805, -3.092) (-19.2832, -3.0811) (-19.2859, -3.0702) (-19.2887, -3.0594) (-19.2916, -3.0486) (-19.2946, -3.0379) (-19.2977, -3.0273) (-19.3008, -3.0167) (-19.3041, -3.0061) (-19.3074, -2.9956) (-19.3108, -2.9852) (-19.3143, -2.9748) (-19.3179, -2.9645) (-19.3216, -2.9542) (-19.3254, -2.944) (-19.3293, -2.9339) (-19.3333, -2.9239) (-19.3374, -2.9139) (-19.3417, -2.9041) (-19.3462, -2.8943) (-19.3507, -2.8846) (-19.3552, -2.8749) (-19.3599, -2.8653) (-19.3646, -2.8558) (-19.3695, -2.8463) (-19.3747, -2.8371) (-19.3792, -2.83) (-19.3827, -2.8248) (-19.3852, -2.8214) (-19.3865, -2.8197) knots -1 -1 -1 -1 -1 -1 -0.98571429 -0.97142857 -0.95714286 -0.94285714 -0.92857143 -0.91428571 -0.9 -0.88571429 -0.87142857 -0.85714286 -0.84285714 -0.82857143 -0.81428571 -0.8 -0.78571429 -0.77142857 -0.75714286 -0.74285714 -0.72857143 -0.71428571 -0.7 -0.68571429 -0.67142857 -0.65714286 -0.64285714 -0.62857143 -0.61428571 -0.6 -0.58571429 -0.57142857 -0.55714286 -0.54285714 -0.52857143 -0.51428571 -0.5 -0.48571429 -0.47142857 -0.45714286 -0.44285714 -0.42857143 -0.41428571 -0.4 -0.38571429 -0.37142857 -0.35714286 -0.34285714 -0.32857143 -0.31428571 -0.3 -0.28571429 -0.27142857 -0.25714286 -0.24285714 -0.22857143 -0.21428571 -0.2 -0.18571429 -0.17142857 -0.15714286 -0.14285714 -0.12857143 -0.11428571 -0.1 -0.08571429 -0.07142857 -0.05714286 -0.04285714 -0.02857143 -0.01428571 0 0 0 0 0 0
  line L27 (-19.3865, -2.8197) -> (-19.4814, -2.693)
  arc A55 (-19.4506, -2.4204) -> (-19.4814, -2.693) centre (-19.3214, -2.5731) ccw
  arc A56 (-19.4506, -2.4204) -> (-19.3071, -2.2912) centre (-21.5, 0) ccw
  arc A57 (-19.0327, -2.289) -> (-19.3071, -2.2912) centre (-19.1688, -2.4356) ccw
  line L28 (-19.0327, -2.289) -> (-18.9167, -2.3967)
  spline S28 degree 5 poles (-18.9167, -2.3967) (-18.9152, -2.3981) (-18.912, -2.4009) (-18.9072, -2.405) (-18.9006, -2.4102) (-18.8919, -2.4164) (-18.8831, -2.4222) (-18.8741, -2.4279) (-18.865, -2.4335) (-18.8559, -2.4391) (-18.8467, -2.4446) (-18.8375, -2.45) (-18.8281, -2.4553) (-18.8186, -2.4605) (-18.8091, -2.4655) (-18.7994, -2.4705) (-18.7897, -2.4753) (-18.7798, -2.48) (-18.7699, -2.4846) (-18.76, -2.4892) (-18.75, -2.4937) (-18.7399, -2.4981) (-18.7297, -2.5025) (-18.7195, -2.5067) (-18.7092, -2.5109) (-18.6989, -2.515) (-18.6885, -2.519) (-18.678, -2.5229) (-18.6675, -2.5267) (-18.657, -2.5305) (-18.6463, -2.5342) (-18.6357, -2.5379) (-18.625, -2.5414) (-18.6142, -2.5449) (-18.6033, -2.5483) (-18.5925, -2.5517) (-18.5815, -2.555) (-18.5706, -2.5582) (-18.5595, -2.5613) (-18.5485, -2.5644) (-18.5374, -2.5674) (-18.5262, -2.5703) (-18.515, -2.5732) (-18.5037, -2.576) (-18.4924, -2.5787) (-18.4811, -2.5814) (-18.4697, -2.584) (-18.4583, -2.5865) (-18.4468, -2.589) (-18.4353, -2.5914) (-18.4238, -2.5937) (-18.4122, -2.596) (-18.4006, -2.5982) (-18.3889, -2.6003) (-18.3772, -2.6024) (-18.3655, -2.6044) (-18.3537, -2.6064) (-18.3419, -2.6083) (-18.3301, -2.6101) (-18.3182, -2.6118) (-18.3063, -2.6135) (-18.2943, -2.6152) (-18.2823, -2.6167) (-18.2703, -2.6182) (-18.2583, -2.6197) (-18.2462, -2.6211) (-18.2341, -2.6224) (-18.2219, -2.6236) (-18.2097, -2.6248) (-18.1975, -2.626) (-18.1853, -2.627) (-18.1754, -2.6278) (-18.1681, -2.6284) (-18.1631, -2.6288) (-18.1607, -2.629) knots 0 0 0 0 0 0 0.01428571 0.02857143 0.04285714 0.05714286 0.07142857 0.08571429 0.1 0.11428571 0.12857143 0.14285714 0.15714286 0.17142857 0.18571429 0.2 0.21428571 0.22857143 0.24285714 0.25714286 0.27142857 0.28571429 0.3 0.31428571 0.32857143 0.34285714 0.35714286 0.37142857 0.38571429 0.4 0.41428571 0.42857143 0.44285714 0.45714286 0.47142857 0.48571429 0.5 0.51428571 0.52857143 0.54285714 0.55714286 0.57142857 0.58571429 0.6 0.61428571 0.62857143 0.64285714 0.65714286 0.67142857 0.68571429 0.7 0.71428571 0.72857143 0.74285714 0.75714286 0.77142857 0.78571429 0.8 0.81428571 0.82857143 0.84285714 0.85714286 0.87142857 0.88571429 0.9 0.91428571 0.92857143 0.94285714 0.95714286 0.97142857 0.98571429 1 1 1 1 1 1
  arc A58 (-18.1607, -2.629) -> (-17.9678, -2.3635) centre (-21.5, 0) ccw
  spline S29 degree 5 poles (-17.9678, -2.3635) (-17.9687, -2.3612) (-17.9706, -2.3566) (-17.9734, -2.3498) (-17.9772, -2.3407) (-17.982, -2.3294) (-17.9869, -2.3181) (-17.9918, -2.3069) (-17.9967, -2.2957) (-18.0017, -2.2846) (-18.0068, -2.2735) (-18.0119, -2.2625) (-18.017, -2.2516) (-18.0222, -2.2406) (-18.0275, -2.2298) (-18.0328, -2.219) (-18.0381, -2.2082) (-18.0435, -2.1975) (-18.0489, -2.1869) (-18.0544, -2.1763) (-18.06, -2.1657) (-18.0656, -2.1552) (-18.0712, -2.1448) (-18.0769, -2.1344) (-18.0826, -2.1241) (-18.0884, -2.1139) (-18.0943, -2.1037) (-18.1001, -2.0935) (-18.1061, -2.0835) (-18.1121, -2.0734) (-18.1181, -2.0635) (-18.1242, -2.0536) (-18.1303, -2.0438) (-18.1365, -2.034) (-18.1428, -2.0243) (-18.1491, -2.0146) (-18.1554, -2.0051) (-18.1618, -1.9955) (-18.1682, -1.9861) (-18.1747, -1.9767) (-18.1813, -1.9674) (-18.1879, -1.9582) (-18.1945, -1.949) (-18.2012, -1.9399) (-18.208, -1.9309) (-18.2148, -1.9219) (-18.2216, -1.913) (-18.2286, -1.9042) (-18.2355, -1.8955) (-18.2425, -1.8868) (-18.2496, -1.8783) (-18.2568, -1.8698) (-18.264, -1.8614) (-18.2712, -1.8531) (-18.2785, -1.8449) (-18.2859, -1.8367) (-18.2933, -1.8287) (-18.3008, -1.8207) (-18.3083, -1.8128) (-18.3159, -1.805) (-18.3236, -1.7973) (-18.3314, -1.7898) (-18.3392, -1.7824) (-18.3471, -1.7751) (-18.3552, -1.768) (-18.3632, -1.761) (-18.3713, -1.754) (-18.3795, -1.7471) (-18.3877, -1.7403) (-18.396, -1.7337) (-18.4045, -1.7274) (-18.4115, -1.7227) (-18.4168, -1.7194) (-18.4205, -1.7173) (-18.4223, -1.7162) knots -1 -1 -1 -1 -1 -1 -0.98571429 -0.97142857 -0.95714286 -0.94285714 -0.92857143 -0.91428571 -0.9 -0.88571429 -0.87142857 -0.85714286 -0.84285714 -0.82857143 -0.81428571 -0.8 -0.78571429 -0.77142857 -0.75714286 -0.74285714 -0.72857143 -0.71428571 -0.7 -0.68571429 -0.67142857 -0.65714286 -0.64285714 -0.62857143 -0.61428571 -0.6 -0.58571429 -0.57142857 -0.55714286 -0.54285714 -0.52857143 -0.51428571 -0.5 -0.48571429 -0.47142857 -0.45714286 -0.44285714 -0.42857143 -0.41428571 -0.4 -0.38571429 -0.37142857 -0.35714286 -0.34285714 -0.32857143 -0.31428571 -0.3 -0.28571429 -0.27142857 -0.25714286 -0.24285714 -0.22857143 -0.21428571 -0.2 -0.18571429 -0.17142857 -0.15714286 -0.14285714 -0.12857143 -0.11428571 -0.1 -0.08571429 -0.07142857 -0.05714286 -0.04285714 -0.02857143 -0.01428571 0 0 0 0 0 0
  line L29 (-18.4223, -1.7162) -> (-18.5606, -1.6392)
  arc A59 (-18.6433, -1.3776) -> (-18.5606, -1.6392) centre (-18.4632, -1.4645) ccw
  circle A60 centre (-21.5, 0) radius 2
  line L30 (-21.5, 0) -> (-21.5, 2)
  circle A61 centre (-21.5, 0) radius 2
  line L31 (-21.5, 0) -> (-22.2, 0)
  line L32 (-22.2, 0) -> (-22.2, 1.8735)
  line L33 (-21.5, 0) -> (-20.8, 0)
  line L34 (-20.8, 0) -> (-20.8, 1.8735)
  line L35 (-21.5, 2) -> (-21.5, 1.35)
  line L36 (-22.2, 1.35) -> (-20.8, 1.35)
  line L37 (-21.5, -0.7) -> (-23.3735, -0.7)
  line L38 (-22.85, -0.7) -> (-22.85, 0.7)
  line L39 (-21.5, 0.7) -> (-23.3735, 0.7)
  line L40 (-20.8, 0) -> (-20.8, -1.8735)
  line L41 (-20.8, -1.35) -> (-22.2, -1.35)
  line L42 (-22.2, 0) -> (-22.2, -1.8735)
  line L43 (-21.5, 0.7) -> (-19.6265, 0.7)
  line L44 (-20.15, 0.7) -> (-20.15, -0.7)
  line L45 (-21.5, -0.7) -> (-19.6265, -0.7)
  dimension "d71" = 0.7
  dimension "d72" = 0.7
  dimension "d73" = 0.65
  dimension "d75" = 360
  constraint coincident A0.centre A2.centre
  constraint coincident A60 L30.end
  constraint vertical L30
  constraint perpendicular L30 L31
  constraint coincident A61 L32.end
  constraint perpendicular L31 L32
  constraint perpendicular L30 L33
  constraint coincident A61 L34.end
  constraint perpendicular L33 L34
  constraint perpendicular L33 L35
  constraint midpoint L35.end L36
  constraint coincident L34 L36.end
  constraint perpendicular L34 L36
  measures "d71" distance of A0.centre L31.end
  measures "d72" distance of A0.centre L33.end
  measures "d73" distance of L30.end L35.end
extrude "Extrude18" add sketch "Sketch26" against normal blind 4 contours A60 A61 L43 L44 L45 | A60 L30 A61 L34 L35 L36 | A60 A61 L40 L41 L42 | A60 L30 A61 L32 L35 L36 | A60 A61 L37 L38 L39 bodies 3
fillet "Fillet9" radius 0.1 8 edges at (-22.2, -1.8735, 2) (-20.8, -1.8735, 2) (-19.6265, -0.7, 2) (-19.6265, 0.7, 2) (-20.8, 1.8735, 2) (-22.2, 1.8735, 2) (-23.3735, 0.7, 2) (-23.3735, -0.7, 2) on bodies 3
fillet "Fillet10" radius 0.1 8 edges at (-20.8, 1.35, 2) (-22.2, 1.35, 2) (-20.15, 0.7, 2) (-20.15, -0.7, 2) (-20.8, -1.35, 2) (-22.2, -1.35, 2) (-22.85, -0.7, 2) (-22.85, 0.7, 2) on bodies 3